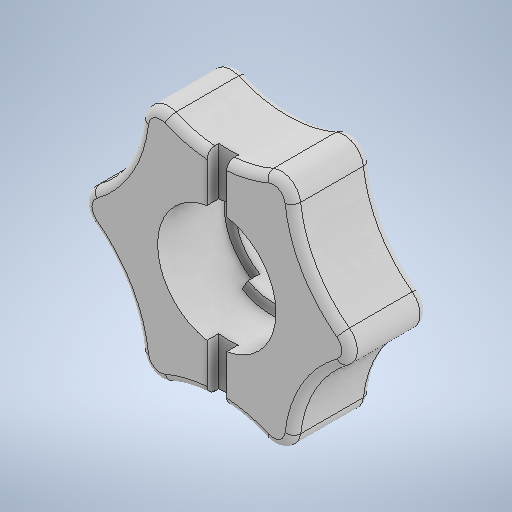
# Autodesk Inventor part: Tool-Lock-Knob
Saved by Autodesk Inventor 2025.3 (Build 293356030, 356C)
## iProperties
Created: 2025-10-10
Part Number: Tool-Lock-Knob
Material: Generic
Document SubType Name: Modeling
Designer: tvoko
Density: 1 g/cm^3
Appearance: Default
Author: tvoko
Autodesk Inventor part; units mm, degrees
ref_plane "YZ Plane" through (0, 0, 0) normal (1, 0, 0) x (0, 1, 0)
ref_plane "XZ Plane" through (0, 0, 0) normal (0, 1, 0) x (-1, 0, 0)
ref_plane "XY Plane" through (0, 0, 0) normal (0, 0, 1) x (1, 0, 0)
sketch "Sketch1" plane through (0, 0, 0) normal (0, 0, 1) x (1, 0, 0)
  circle A0 centre (0, 0) radius 15.1
  line L0 (-17.3205, -30) -> (-34.641, 0) construction
  line L1 (-34.641, 0) -> (-17.3205, 30) construction
  line L2 (-17.3205, 30) -> (17.3205, 30) construction
  line L3 (17.3205, 30) -> (34.641, 0) construction
  line L4 (34.641, 0) -> (17.3205, -30) construction
  line L5 (17.3205, -30) -> (-17.3205, -30) construction
  arc A1 (14.4338, 30) -> (12.4414, 29.5859) centre (14.4338, 25) ccw
  arc A2 (-12.4414, 29.5859) -> (-18.7639, 27.5) centre (-14.4338, 25) ccw
  arc A3 (-12.4414, 29.5859) -> (12.4414, 29.5859) centre (0, 58.2222) ccw
  circle A4 centre (0, 0) radius 27 construction
  arc A5 (-31.8428, 4.0184) -> (-19.4014, 25.5675) centre (-50.4219, 29.1111) ccw
  arc A6 (-31.8428, 4.0184) -> (-33.1976, -2.5) centre (-28.8675, 0) ccw
  arc A7 (-18.7639, 27.5) -> (-19.4014, 25.5675) centre (-14.4338, 25) ccw
  arc A8 (-19.4014, -25.5675) -> (-31.8428, -4.0184) centre (-50.4219, -29.1111) ccw
  arc A9 (-19.4014, -25.5675) -> (-14.4338, -30) centre (-14.4338, -25) ccw
  arc A10 (-33.1976, -2.5) -> (-31.8428, -4.0184) centre (-28.8675, 0) ccw
  arc A11 (12.4414, -29.5859) -> (-12.4414, -29.5859) centre (0, -58.2222) ccw
  arc A12 (12.4414, -29.5859) -> (18.7639, -27.5) centre (14.4338, -25) ccw
  arc A13 (-14.4338, -30) -> (-12.4414, -29.5859) centre (-14.4338, -25) ccw
  arc A14 (31.8428, -4.0184) -> (19.4014, -25.5675) centre (50.4219, -29.1111) ccw
  arc A15 (31.8428, -4.0184) -> (33.1976, 2.5) centre (28.8675, 0) ccw
  arc A16 (18.7639, -27.5) -> (19.4014, -25.5675) centre (14.4338, -25) ccw
  arc A17 (19.4014, 25.5675) -> (31.8428, 4.0184) centre (50.4219, 29.1111) ccw
  arc A18 (19.4014, 25.5675) -> (14.4338, 30) centre (14.4338, 25) ccw
  arc A19 (33.1976, 2.5) -> (31.8428, 4.0184) centre (28.8675, 0) ccw
  circle A20 centre (0, 0) radius 12.1
  line L6 (0, 15.1) -> (0, -15.1) construction
  line L7 (-7.55, 13.077) -> (7.55, -13.077)
  line L8 (7.55, 13.077) -> (-7.55, -13.077)
  point P0 (14.4338, 30)
  point P1 (-33.1976, -2.5)
  point P2 (-14.4338, -30)
  point P3 (18.7639, -27.5)
  point P4 (33.1976, 2.5)
  point P5 (-15.1, 0)
  point P6 (15.1, 0)
  point P7 (0, 12.1)
  point P8 (0, -12.1)
  point P9 (-6.05, -10.4789)
  point P10 (7.55, -13.077)
  point P11 (6.05, -10.4789)
  point P12 (6.05, 10.4789)
  point P13 (-6.05, 10.4789)
  dimension "d0" = 30.2
  dimension "d1" = 60
  dimension "d4" = 5
  dimension "d5" = 54
  dimension "d8" = 360
  dimension "d10" = 3
  dimension "d13" = 60
  dimension "d14" = 30
  constraints: 48 point on circle, 20 centre point, 18 end point, 7 tangent, 4 coincident, 3 midpoint, 2 point on line, 1 equal radius, 1 horizontal, 1 vertical, 83 other
  measures "d1" distance between parallel lines of L5 L2
  measures "d4" radius of A2
  measures "d5" diameter of A4
  measures "d13" angle of L8 L7
  measures "d14" angle of L6 L8
extrude "Extrusion1" add sketch "Sketch1" along normal blind 20
extrude "Extrusion2" add sketch "Sketch1" along normal blind 3 contours A0 L7 A20 L8 | L8 A20 L7 A0 | A0 L8 A20 L7 | L7 A20 L8 A0
extrude "Extrusion3" add sketch "Sketch1" along normal blind 6 contours L8 A20 L7 A0 | A0 L8 A20 L7 picked at (6.0887, 12.639) picked at (-6.0887, -12.639)
sketch "Sketch2" plane through (0, 0, 20) normal (0, 0, 1) x (1, 0, 0)
  arc A0 (19.4014, 25.5675) -> (12.4414, 29.5859) centre (14.4338, 25) ccw projected
  arc A1 (-12.4414, 29.5859) -> (12.4414, 29.5859) centre (0, 58.2222) ccw projected
  arc A2 (-12.4414, 29.5859) -> (-19.4014, 25.5675) centre (-14.4338, 25) ccw projected
  arc A3 (-31.8428, 4.0184) -> (-19.4014, 25.5675) centre (-50.4219, 29.1111) ccw projected
  arc A4 (-31.8428, 4.0184) -> (-31.8428, -4.0184) centre (-28.8675, 0) ccw projected
  arc A5 (-19.4014, -25.5675) -> (-31.8428, -4.0184) centre (-50.4219, -29.1111) ccw projected
  arc A6 (-19.4014, -25.5675) -> (-12.4414, -29.5859) centre (-14.4338, -25) ccw projected
  arc A7 (12.4414, -29.5859) -> (-12.4414, -29.5859) centre (0, -58.2222) ccw projected
  arc A8 (12.4414, -29.5859) -> (19.4014, -25.5675) centre (14.4338, -25) ccw projected
  arc A9 (31.8428, -4.0184) -> (19.4014, -25.5675) centre (50.4219, -29.1111) ccw projected
  arc A10 (31.8428, -4.0184) -> (31.8428, 4.0184) centre (28.8675, 0) ccw projected
  arc A11 (19.4014, 25.5675) -> (31.8428, 4.0184) centre (50.4219, 29.1111) ccw projected
  circle A12 centre (0, 0) radius 15.1 projected
  line L0 (0, 27) -> (0, -27) construction
  line L1 (-2.5, 27.1002) -> (-2.5, -27.1002)
  line L2 (2.5, 27.1002) -> (2.5, -27.1002)
  line L3 (-2.5, 0) -> (2.5, 0) construction
  point P0 (0, 0)
  point P1 (2.5, -14.8916)
  point P2 (-2.5, -14.8916)
  point P3 (2.5, 14.8916)
  point P4 (-2.5, 14.8916)
  dimension "d17" = 5
  constraints: 8 end point, 6 point on circle, 4 midpoint, 2 perpendicular, 1 vertical
  measures "d17" distance between parallel lines of L1 L2
extrude "Extrusion4" cut sketch "Sketch2" against normal blind 3 contours L2 A12 L1 A1 | L2 A7 L1 A12
ref_plane "Work Plane1" through (0, 0, 0) normal (1, 0, 0) x (0, 0, 1)
sketch "Sketch3" plane through (0, 0, 0) normal (1, 0, 0) x (0, 0, 1)
  line L0 (17, 27) -> (17, 15.1) projected
  line L1 (17, 15.1) -> (6, 15.1) projected
  line L2 (6, 15.1) -> (6, 12.1) projected
  line L3 (6, 12.1) -> (0, 12.1) projected
  line L4 (0, 12.1) -> (0, 27) projected
  line L5 (0, 27) -> (17, 27) projected
  line L6 (17, -15.1) -> (17, -27) projected
  line L7 (17, -27) -> (0, -27) projected
  line L8 (0, -27) -> (0, -12.1) projected
  line L9 (0, -12.1) -> (6, -12.1) projected
  line L10 (6, -12.1) -> (6, -15.1) projected
  line L11 (6, -15.1) -> (17, -15.1) projected
  point P0 (0, 0)
ref_plane "Work Plane2" through (0, 15.1, 6) normal (0, 1, 0) x (-1, 0, 0)
sketch "Sketch4" plane through (0, 15.1, 6) normal (0, 1, 0) x (-1, 0, 0)
  line L0 (-2.829, 5) -> (-1.4145, 7.45)
  line L1 (-1.4145, 7.45) -> (1.4145, 7.45)
  line L2 (1.4145, 7.45) -> (2.829, 5)
  line L3 (2.829, 5) -> (1.4145, 2.55)
  line L4 (1.4145, 2.55) -> (-1.4145, 2.55)
  line L5 (-1.4145, 2.55) -> (-2.829, 5)
  line L6 (-7.55, 0) -> (7.55, 0) projected
  line L7 (0, 0) -> (0, 11) projected
  point P0 (0, -6)
  point P1 (0, 5)
  point P2 (0, 0)
  dimension "d21" = 5
  dimension "d22" = 4.9
  constraints: 12 end point, 1 midpoint, 1 parallel, 1 point on line, 13 other
  measures "d21" distance of point (0, 0) point (0, 5)
  measures "d22" distance between parallel lines of L4 L1
extrude "Extrusion5" cut sketch "Sketch4" along normal mid plane 2.5
chamfer "Chamfer1" distance 0.5 angle 45 6 edges at (-2.1241, 14.9499, 9.7791) (-2.1241, 14.9499, 12.2209) (0, 15.1, 13.45) (2.1241, 14.9499, 12.2209) (2.1241, 14.9499, 9.7791) (0, 15.1, 8.55)
fillet "Fillet1" radius 2 26 edges at (16.9338, 29.3301, 0) (0, 27, 0) (-16.9338, 29.3301, 0) (-23.3827, 13.5, 0) (-33.8675, 0, 0) (-23.3827, -13.5, 0) (-16.9338, -29.3301, 0) (0, -27, 0) (16.9338, -29.3301, 0) (23.3827, -13.5, 0) (33.8675, 0, 0) (23.3827, 13.5, 0) (16.9338, 29.3301, 20) (7.5734, 27.9324, 20) (33.8675, 0, 20) (23.3827, -13.5, 20) (16.9338, -29.3301, 20) (7.5734, -27.9324, 20) (23.3827, 13.5, 20) (-16.9338, 29.3301, 20) (-23.3827, 13.5, 20) (-33.8675, 0, 20) (-23.3827, -13.5, 20) (-16.9338, -29.3301, 20) (-7.5734, -27.9324, 20) (-7.5734, 27.9324, 20)
body "Solid1"
